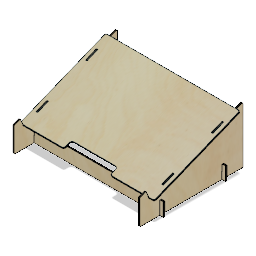
876543210 fótastandur v1 (Autodesk Fusion 360 design; units mm, degrees)
Autodesk Fusion 360 part; units mm, degrees
sketch "Sketch1" plane through (0, 0, 0) normal (1, 0, 0) x (0, 0, -1)
  line L0 (0, 0) -> (0, 55)
  line L1 (0, 55) -> (13.9078, 60.6191)
  line L2 (13.9078, 60.6191) -> (21.4942, 41.8419)
  line L3 (21.4942, 41.8419) -> (225, 124.0636)
  line L4 (225, 124.0636) -> (225, 0)
  line L5 (225, 0) -> (0, 0)
  dimension "d1" = 225
  dimension "d2" = 55
  dimension "d3" = 15
  dimension "d4" = 22
  constraint coincident L0.start L5.end
  constraint vertical L0
  constraint vertical L4
  constraint perpendicular L0 L5
  constraint parallel L1 L3
  constraint perpendicular L2 L3
  measures "d1" distance of L0.start L4.end
  measures "d2" distance of L0.start L0.end
  measures "d3" distance of L0.end L1.end
  measures "d4" angle of L3 L5
extrude "Extrude1" add sketch "Sketch1" along normal blind 2.9 makes body 1
fillet "Fillet1" radius 3 4 edges at (1.45, 55, 0) (1.45, 0, 0) (1.45, 124.0636, -225) (1.45, 0, -225) on bodies 1
fillet "Fillet2" radius 2 2 edges at (1.45, 60.6191, -13.9078) (1.45, 41.8419, -21.4942) on bodies 1
copy_body "Body->Comp2" bodies 1 removing the originals makes body 2 in component "fótur"
sketch "Sketch3" plane through (0, 28.5047, 11.5166) normal (0, 0.927184, 0.374607) x (1, 0, 0)
  line L0 (47.7026, 37.6034) -> (50.6026, 37.6034)
  line L1 (50.6026, 37.6034) -> (50.6026, 250.6437)
  line L2 (50.6026, 250.6437) -> (47.7026, 250.6437)
  line L3 (47.7026, 250.6437) -> (47.7026, 37.6034)
  line L4 (-225.1974, 37.6034) -> (-222.2974, 37.6034)
  line L5 (-222.2974, 37.6034) -> (-222.2974, 250.6437)
  line L6 (-222.2974, 250.6437) -> (-225.1974, 250.6437)
  line L7 (-225.1974, 250.6437) -> (-225.1974, 37.6034)
  line L8 (-233.1974, 238.6437) -> (58.6026, 238.6437)
  line L9 (58.6026, 238.6437) -> (58.6026, 37.6034)
  line L10 (58.6026, 37.6034) -> (-233.1974, 37.6034)
  line L11 (-233.1974, 37.6034) -> (-233.1974, 238.6437)
  line L12 (-87.2974, 238.6437) -> (-87.2974, 37.6034) construction
  line L13 (-233.1974, 138.1235) -> (58.6026, 138.1235) construction
  line L14 (-225.1974, 208.6437) -> (-222.2974, 208.6437)
  line L15 (-222.2974, 208.6437) -> (-222.2974, 183.6437)
  line L16 (-222.2974, 183.6437) -> (-225.1974, 183.6437)
  line L17 (-225.1974, 183.6437) -> (-225.1974, 208.6437)
  line L18 (-225.1974, 205.8348) -> (-225.1974, 2.7816)
  line L19 (-222.2974, 2.7816) -> (-222.2974, 205.8348)
  line L20 (50.6026, 208.6437) -> (47.7026, 208.6437)
  line L21 (47.7026, 183.6437) -> (50.6026, 183.6437)
  line L22 (50.6026, 183.6437) -> (50.6026, 208.6437)
  line L23 (47.7026, 208.6437) -> (47.7026, 183.6437)
  line L24 (-225.1974, 67.6034) -> (-222.2974, 67.6034)
  line L25 (-222.2974, 92.6034) -> (-225.1974, 92.6034)
  line L26 (-222.2974, 67.6034) -> (-222.2974, 92.6034)
  line L27 (-225.1974, 92.6034) -> (-225.1974, 67.6034)
  line L28 (50.6026, 67.6034) -> (47.7026, 67.6034)
  line L29 (47.7026, 67.6034) -> (47.7026, 92.6034)
  line L30 (50.6026, 92.6034) -> (50.6026, 67.6034)
  line L31 (47.7026, 92.6034) -> (50.6026, 92.6034)
  dimension "d42" = 8
  dimension "d43" = 8
  dimension "d44" = 12
  dimension "d45" = 25
  dimension "d46" = 30
  constraint horizontal L8
  constraint vertical L9
  constraint horizontal L10
  constraint vertical L11
  constraint collinear L0 L10
  constraint midpoint L8 L12.start
  constraint midpoint L10 L12.end
  constraint midpoint L11 L13.start
  constraint midpoint L9 L13.end
  constraint horizontal L14
  constraint vertical L15
  constraint horizontal L16
  constraint vertical L17
  constraint coincident L5 L15.end
  constraint coincident L7 L14.start
  constraint symmetric L12 L14.start L20.start
  constraint symmetric L12 L14.end L20.end
  constraint symmetric L12 L15.end L21.start
  constraint symmetric L12 L16.end L21.end
  constraint symmetric L13 L14.start L24.start
  constraint symmetric L13 L14.end L24.end
  constraint symmetric L13 L15.end L25.start
  constraint symmetric L13 L16.end L25.end
  constraint symmetric L13 L20.start L28.start
  constraint symmetric L13 L20.end L28.end
  constraint symmetric L13 L21.start L29.end
  constraint symmetric L13 L21.end L30.start
  measures "d42" distance of L7 L11
  measures "d43" distance of L1 L9
  measures "d44" distance of L1.end L8
  measures "d45" distance of L14 L16
  measures "d46" distance of L8 L14
extrude "Extrude1'" add sketch "Sketch3" against normal blind 2.9 separate body contours L0 L1 L3 L10 L28 | L3 L5 L8 L10 L15 L19 L23 L26 L29 | L1 L8 L9 L10 L22 L30 | L4 L5 L7 L10 L18 L19 L24 | L1 L3 L21 L31 | L7 L8 L10 L11 L17 L18 L27 | L5 L7 L16 L18 L19 L25 | L1 L3 L8 L20 | L5 L7 L8 L14 makes body 3 in component "Top"
combine "Combine1" operation cut target body 2 tool bodies 3 body 3 seen with x (1, 0, 0) y (0, 1, 0) z (0, 0, 1) at (-47.7026, 0, 0) keep tools in component "fótur"
combine "Combine2" operation cut target body 2 tool bodies 3 body 3 seen with x (1, 0, 0) y (0, 1, 0) z (0, 0, 1) at (225.1974, 0, 0) keep tools in component "fótur"
fillet "Fillet1'" radius 4 4 edges at (58.6026, 41.2467, -23.8918) (58.6026, 116.5577, -210.2932) (-233.1974, 116.5577, -210.2932) (-233.1974, 41.2467, -23.8918) on bodies 3 in component "Top"
fillet "Fillet1''" radius 1 5 edges at (1.45, 42.5911, -23.3486) (1.45, 53.8293, -51.1641) (1.45, 63.1945, -74.3437) (1.45, 97.2988, -158.7549) (1.45, 106.664, -181.9345) on bodies 2 in component "fótur"
ref_plane "WorkPlane1" through (49.1526, 61.3079, -180) normal (0, 0, -1) x (0, 1, 0)
sketch "Sketch5" plane through (50.8776, 60.8254, -180) normal (0, 0, -1) x (1, 0, 0)
  line L0 (-273.175, -45.057) -> (-273.175, 60.8254)
  line L1 (-273.175, 60.8254) -> (-276.075, 60.8254)
  line L2 (-276.075, 60.8254) -> (-276.075, -45.057)
  line L3 (-0.275, -45.057) -> (-0.275, 60.8254)
  line L4 (-0.275, 60.8254) -> (-3.175, 60.8254)
  line L5 (-3.175, 60.8254) -> (-3.175, -45.057)
  line L6 (7.725, 30.8254) -> (-284.075, 30.8254)
  line L7 (-284.075, 30.8254) -> (-284.075, 60.8254)
  line L8 (-284.075, 60.8254) -> (7.725, 60.8254)
  line L9 (7.725, 60.8254) -> (7.725, 30.8254)
  line L10 (7.725, -52.8895) -> (7.725, 19.4247)
  line L11 (-284.075, 19.4247) -> (-284.075, -52.8895)
  line L12 (-0.275, 30.8254) -> (-3.175, 30.8254)
  line L13 (-3.175, 30.8254) -> (-3.175, 45.8254)
  line L14 (-3.175, 45.8254) -> (-0.275, 45.8254)
  line L15 (-0.275, 45.8254) -> (-0.275, 30.8254)
  line L16 (-276.075, 30.8254) -> (-273.175, 30.8254)
  line L17 (-273.175, 30.8254) -> (-273.175, 45.8254)
  line L18 (-273.175, 45.8254) -> (-276.075, 45.8254)
  line L19 (-276.075, 45.8254) -> (-276.075, 30.8254)
  line L20 (-276.075, -45.057) -> (-273.175, -45.057)
  line L21 (-3.175, -45.057) -> (-0.275, -45.057)
  dimension "d55" = 30
  dimension "d56" = 15
  dimension "d57" = 15
  constraint horizontal L6
  constraint vertical L7
  constraint horizontal L8
  constraint vertical L9
  constraint collinear L1 L8
  constraint collinear L9 L10
  constraint collinear L7 L11
  constraint horizontal L12
  constraint vertical L13
  constraint horizontal L14
  constraint vertical L15
  constraint coincident L5 L13.end
  constraint coincident L6 L12.start
  constraint coincident L3 L12.start
  constraint horizontal L16
  constraint vertical L17
  constraint horizontal L18
  constraint vertical L19
  constraint coincident L0 L17.end
  constraint coincident L2 L16.start
  constraint coincident L6 L16.start
  measures "d55" distance of L6 L8
  measures "d56" distance of L6 L14
  measures "d57" distance of L6 L18
extrude "Extrude2" add sketch "Sketch5" along normal mid plane 2.9 separate body contours L0 L5 L6 L8 L13 L17 | L0 L1 L2 L8 L18 | L2 L6 L7 L8 L19 | L3 L4 L5 L8 L14 | L3 L6 L8 L9 L15 makes body 4
ref_plane "WorkPlane2" through (49.1526, 27.9882, -112.5) normal (0, 0, 1) x (0, -1, 0)
mirror "Mirror1" about plane through (49.1526, 27.9882, -112.5) normal (0, 0, 1) of bodies 4 makes body 5
combine "Combine3" operation cut target body 2 tool bodies 4 5 body 4 seen with x (1, 0, 0) y (0, 1, 0) z (0, 0, 1) at (-47.7026, 0, 0) body 5 seen with x (1, 0, 0) y (0, 1, 0) z (0, 0, 1) at (-47.7026, 0, 0) keep tools in component "fótur"
combine "Combine4" operation cut target body 2 tool bodies 4 5 body 4 seen with x (1, 0, 0) y (0, 1, 0) z (0, 0, 1) at (225.1974, 0, 0) body 5 seen with x (1, 0, 0) y (0, 1, 0) z (0, 0, 1) at (225.1974, 0, 0) keep tools in component "fótur"
fillet "Fillet3" radius 1 12 edges at (50.6026, 30, -180) (47.7026, 30, -180) (58.6026, 30, -180) (-222.2974, 30, -180) (-225.1974, 30, -180) (-233.1974, 30, -180) (50.6026, 30, -45) (47.7026, 30, -45) (-222.2974, 30, -45) (-225.1974, 30, -45) (-233.1974, 30, -45) (58.6026, 30, -45) on bodies 4 5
fillet "Fillet2'" radius 1 4 edges at (1.45, 0, -43.55) (1.45, 0, -46.45) (1.45, 0, -178.55) (1.45, 0, -181.45) on bodies 2 in component "fótur"
sketch "Sketch6" plane through (0, 28.5047, 11.5166) normal (0, 0.927184, 0.374607) x (1, 0, 0)
  arc A0 (-233.1974, 41.6034) -> (-229.1974, 37.6034) centre (-229.1974, 41.6034) ccw
  line L0 (-229.1974, 37.6034) -> (54.6026, 37.6034)
  arc A1 (54.6026, 37.6034) -> (58.6026, 41.6034) centre (54.6026, 41.6034) ccw
  line L1 (58.6026, 41.6034) -> (58.6026, 234.6437)
  arc A2 (58.6026, 234.6437) -> (54.6026, 238.6437) centre (54.6026, 234.6437) ccw
  line L2 (54.6026, 238.6437) -> (-229.1974, 238.6437)
  arc A3 (-229.1974, 238.6437) -> (-233.1974, 234.6437) centre (-229.1974, 234.6437) ccw
  line L3 (-233.1974, 234.6437) -> (-233.1974, 41.6034)
  line L4 (47.7026, 67.6034) -> (47.7026, 92.6034)
  line L5 (47.7026, 92.6034) -> (50.6026, 92.6034)
  line L6 (50.6026, 92.6034) -> (50.6026, 67.6034)
  line L7 (50.6026, 67.6034) -> (47.7026, 67.6034)
  line L8 (-225.1974, 183.6437) -> (-225.1974, 208.6437)
  line L9 (-225.1974, 208.6437) -> (-222.2974, 208.6437)
  line L10 (-222.2974, 208.6437) -> (-222.2974, 183.6437)
  line L11 (-222.2974, 183.6437) -> (-225.1974, 183.6437)
  line L12 (-225.1974, 67.6034) -> (-225.1974, 92.6034)
  line L13 (-225.1974, 92.6034) -> (-222.2974, 92.6034)
  line L14 (-222.2974, 92.6034) -> (-222.2974, 67.6034)
  line L15 (-222.2974, 67.6034) -> (-225.1974, 67.6034)
  line L16 (47.7026, 183.6437) -> (47.7026, 208.6437)
  line L17 (47.7026, 208.6437) -> (50.6026, 208.6437)
  line L18 (50.6026, 208.6437) -> (50.6026, 183.6437)
  line L19 (50.6026, 183.6437) -> (47.7026, 183.6437)
  line L20 (-229.1974, 238.6437) -> (54.6026, 238.6437)
  line L21 (54.6026, 37.6034) -> (-229.1974, 37.6034)
  line L22 (-137.2974, 55.1034) -> (-37.2974, 55.1034)
  line L23 (-37.2974, 55.1034) -> (-37.2974, 20.1034)
  line L24 (-37.2974, 20.1034) -> (-137.2974, 20.1034)
  line L25 (-137.2974, 20.1034) -> (-137.2974, 55.1034)
  line L26 (-137.2974, 55.1034) -> (-37.2974, 20.1034) construction
  line L27 (-37.2974, 55.1034) -> (-137.2974, 20.1034) construction
  point P0 (-87.2974, 37.6034)
  dimension "d64" = 100
  dimension "d65" = 35
  constraint perpendicular L22 L23
  constraint parallel L22 L24
  constraint parallel L23 L25
  constraint horizontal L22
  constraint coincident L26 P0
  constraint coincident L27 P0
  constraint midpoint L21 P0
  measures "d64" distance of L23.end L24.end
  measures "d65" distance of L22.end L23.end
extrude "Extrude2'" cut sketch "Sketch6" against normal up to surface (2.9 mm away) contours L0 L21 L22 L23 L25 bodies 3 in component "Top"
fillet "Fillet2''" radius 5 4 edges at (-37.2974, 47.8023, -40.1175) (-37.2974, 41.2467, -23.8918) (-137.2974, 47.8023, -40.1175) (-137.2974, 41.2467, -23.8918) on bodies 3 in component "Top"
sketch "Sketch10" plane through (50.6026, 0, 0) normal (1, 0, 0) x (0, 0, -1)
  arc A0 (181.45, 1) -> (182.45, 0) centre (182.45, 1) ccw
  line L0 (182.45, 0) -> (222, 0)
  arc A1 (222, 0) -> (225, 3) centre (222, 3) ccw
  line L1 (225, 3) -> (225, 119.6159)
  arc A2 (225, 119.6159) -> (220.8762, 122.3974) centre (222, 119.6159) ccw
  line L2 (220.8762, 122.3974) -> (209.75, 117.9022)
  line L3 (209.75, 117.9022) -> (210.8363, 115.2133)
  line L4 (210.8363, 115.2133) -> (183.0208, 103.9751)
  line L5 (183.0208, 103.9751) -> (182.3091, 105.7368)
  arc A3 (182.3091, 105.7368) -> (181.0073, 106.2894) centre (181.3819, 105.3622) ccw
  line L6 (181.0073, 106.2894) -> (159.682, 97.6734)
  arc A4 (159.682, 97.6734) -> (159.1295, 96.3716) centre (160.0567, 96.7462) ccw
  line L7 (159.1295, 96.3716) -> (159.8412, 94.61)
  line L8 (159.8412, 94.61) -> (75.4301, 60.5056)
  line L9 (75.4301, 60.5056) -> (74.7183, 62.2673)
  arc A5 (74.7183, 62.2673) -> (73.4165, 62.8199) centre (73.7911, 61.8927) ccw
  line L10 (73.4165, 62.8199) -> (52.0913, 54.2039)
  arc A6 (52.0913, 54.2039) -> (51.5387, 52.9021) centre (52.4659, 53.2767) ccw
  line L11 (51.5387, 52.9021) -> (52.2505, 51.1405)
  line L12 (52.2505, 51.1405) -> (24.435, 39.9023)
  line L13 (24.435, 39.9023) -> (23.6589, 41.823)
  arc A7 (23.6589, 41.823) -> (22.6876, 42.4474) centre (22.7318, 41.4484) ccw
  arc A8 (20.745, 43.6963) -> (22.6876, 42.4474) centre (22.5994, 44.4455) ccw
  line L14 (20.745, 43.6963) -> (14.657, 58.7647)
  arc A9 (14.657, 58.7647) -> (12.0534, 59.8699) centre (12.8026, 58.0155) ccw
  line L15 (12.0534, 59.8699) -> (1.8762, 55.758)
  arc A10 (1.8762, 55.758) -> (0, 52.9765) centre (3, 52.9765) ccw
  line L16 (0, 52.9765) -> (0, 3)
  arc A11 (0, 3) -> (3, 0) centre (3, 3) ccw
  line L17 (3, 0) -> (42.55, 0)
  arc A12 (42.55, 0) -> (43.55, 1) centre (42.55, 1) ccw
  line L18 (43.55, 1) -> (43.55, 15)
  line L19 (43.55, 15) -> (46.45, 15)
  line L20 (46.45, 15) -> (46.45, 1)
  arc A13 (46.45, 1) -> (47.45, 0) centre (47.45, 1) ccw
  line L21 (47.45, 0) -> (177.55, 0)
  arc A14 (177.55, 0) -> (178.55, 1) centre (177.55, 1) ccw
  line L22 (178.55, 1) -> (178.55, 15)
  line L23 (178.55, 15) -> (181.45, 15)
  line L24 (181.45, 15) -> (181.45, 1)
sketch "Top_DXF" plane through (0, 28.5047, 11.5166) normal (0, 0.927184, 0.374607) x (1, 0, 0)
  line L0 (47.7026, 67.6034) -> (47.7026, 92.6034)
  line L1 (47.7026, 92.6034) -> (50.6026, 92.6034)
  line L2 (50.6026, 92.6034) -> (50.6026, 67.6034)
  line L3 (50.6026, 67.6034) -> (47.7026, 67.6034)
  line L4 (-225.1974, 183.6437) -> (-225.1974, 208.6437)
  line L5 (-225.1974, 208.6437) -> (-222.2974, 208.6437)
  line L6 (-222.2974, 208.6437) -> (-222.2974, 183.6437)
  line L7 (-222.2974, 183.6437) -> (-225.1974, 183.6437)
  line L8 (-225.1974, 67.6034) -> (-225.1974, 92.6034)
  line L9 (-225.1974, 92.6034) -> (-222.2974, 92.6034)
  line L10 (-222.2974, 92.6034) -> (-222.2974, 67.6034)
  line L11 (-222.2974, 67.6034) -> (-225.1974, 67.6034)
  line L12 (47.7026, 183.6437) -> (47.7026, 208.6437)
  line L13 (47.7026, 208.6437) -> (50.6026, 208.6437)
  line L14 (50.6026, 208.6437) -> (50.6026, 183.6437)
  line L15 (50.6026, 183.6437) -> (47.7026, 183.6437)
  arc A0 (-142.2974, 37.6034) -> (-137.2974, 42.6034) centre (-142.2974, 42.6034) ccw
  line L16 (-137.2974, 42.6034) -> (-137.2974, 50.1034)
  arc A1 (-132.2974, 55.1034) -> (-137.2974, 50.1034) centre (-132.2974, 50.1034) ccw
  line L17 (-132.2974, 55.1034) -> (-42.2974, 55.1034)
  arc A2 (-37.2974, 50.1034) -> (-42.2974, 55.1034) centre (-42.2974, 50.1034) ccw
  line L18 (-37.2974, 50.1034) -> (-37.2974, 42.6034)
  arc A3 (-37.2974, 42.6034) -> (-32.2974, 37.6034) centre (-32.2974, 42.6034) ccw
  line L19 (-32.2974, 37.6034) -> (54.6026, 37.6034)
  arc A4 (54.6026, 37.6034) -> (58.6026, 41.6034) centre (54.6026, 41.6034) ccw
  line L20 (58.6026, 41.6034) -> (58.6026, 234.6437)
  arc A5 (58.6026, 234.6437) -> (54.6026, 238.6437) centre (54.6026, 234.6437) ccw
  line L21 (54.6026, 238.6437) -> (-229.1974, 238.6437)
  arc A6 (-229.1974, 238.6437) -> (-233.1974, 234.6437) centre (-229.1974, 234.6437) ccw
  line L22 (-233.1974, 234.6437) -> (-233.1974, 41.6034)
  arc A7 (-233.1974, 41.6034) -> (-229.1974, 37.6034) centre (-229.1974, 41.6034) ccw
  line L23 (-229.1974, 37.6034) -> (-142.2974, 37.6034)
sketch "Support_DXF" plane through (0, 0, -43.55) normal (0, 0, 1) x (1, 0, 0)
  arc A0 (58.6026, 29) -> (57.6026, 30) centre (57.6026, 29) ccw
  line L0 (57.6026, 30) -> (51.6026, 30)
  arc A1 (51.6026, 30) -> (50.6026, 29) centre (51.6026, 29) ccw
  line L1 (50.6026, 29) -> (50.6026, 15)
  line L2 (50.6026, 15) -> (47.7026, 15)
  line L3 (47.7026, 15) -> (47.7026, 29)
  arc A2 (47.7026, 29) -> (46.7026, 30) centre (46.7026, 29) ccw
  line L4 (46.7026, 30) -> (-221.2974, 30)
  arc A3 (-221.2974, 30) -> (-222.2974, 29) centre (-221.2974, 29) ccw
  line L5 (-222.2974, 29) -> (-222.2974, 15)
  line L6 (-222.2974, 15) -> (-225.1974, 15)
  line L7 (-225.1974, 15) -> (-225.1974, 29)
  arc A4 (-225.1974, 29) -> (-226.1974, 30) centre (-226.1974, 29) ccw
  line L8 (-226.1974, 30) -> (-232.1974, 30)
  arc A5 (-232.1974, 30) -> (-233.1974, 29) centre (-232.1974, 29) ccw
  line L9 (-233.1974, 29) -> (-233.1974, 0)
  line L10 (-233.1974, 0) -> (58.6026, 0)
  line L11 (58.6026, 0) -> (58.6026, 29)
sketch "Leg_DXF" plane through (50.6026, 0, 0) normal (1, 0, 0) x (0, 0, -1)
  arc A0 (181.45, 1) -> (182.45, 0) centre (182.45, 1) ccw
  line L0 (182.45, 0) -> (222, 0)
  arc A1 (222, 0) -> (225, 3) centre (222, 3) ccw
  line L1 (225, 3) -> (225, 119.6159)
  arc A2 (225, 119.6159) -> (220.8762, 122.3974) centre (222, 119.6159) ccw
  line L2 (220.8762, 122.3974) -> (209.75, 117.9022)
  line L3 (209.75, 117.9022) -> (210.8363, 115.2133)
  line L4 (210.8363, 115.2133) -> (183.0208, 103.9751)
  line L5 (183.0208, 103.9751) -> (182.3091, 105.7368)
  arc A3 (182.3091, 105.7368) -> (181.0073, 106.2894) centre (181.3819, 105.3622) ccw
  line L6 (181.0073, 106.2894) -> (159.682, 97.6734)
  arc A4 (159.682, 97.6734) -> (159.1295, 96.3716) centre (160.0567, 96.7462) ccw
  line L7 (159.1295, 96.3716) -> (159.8412, 94.61)
  line L8 (159.8412, 94.61) -> (75.4301, 60.5056)
  line L9 (75.4301, 60.5056) -> (74.7183, 62.2673)
  arc A5 (74.7183, 62.2673) -> (73.4165, 62.8199) centre (73.7911, 61.8927) ccw
  line L10 (73.4165, 62.8199) -> (52.0913, 54.2039)
  arc A6 (52.0913, 54.2039) -> (51.5387, 52.9021) centre (52.4659, 53.2767) ccw
  line L11 (51.5387, 52.9021) -> (52.2505, 51.1405)
  line L12 (52.2505, 51.1405) -> (24.435, 39.9023)
  line L13 (24.435, 39.9023) -> (23.6589, 41.823)
  arc A7 (23.6589, 41.823) -> (22.6876, 42.4474) centre (22.7318, 41.4484) ccw
  arc A8 (20.745, 43.6963) -> (22.6876, 42.4474) centre (22.5994, 44.4455) ccw
  line L14 (20.745, 43.6963) -> (14.657, 58.7647)
  arc A9 (14.657, 58.7647) -> (12.0534, 59.8699) centre (12.8026, 58.0155) ccw
  line L15 (12.0534, 59.8699) -> (1.8762, 55.758)
  arc A10 (1.8762, 55.758) -> (0, 52.9765) centre (3, 52.9765) ccw
  line L16 (0, 52.9765) -> (0, 3)
  arc A11 (0, 3) -> (3, 0) centre (3, 3) ccw
  line L17 (3, 0) -> (42.55, 0)
  arc A12 (42.55, 0) -> (43.55, 1) centre (42.55, 1) ccw
  line L18 (43.55, 1) -> (43.55, 15)
  line L19 (43.55, 15) -> (46.45, 15)
  line L20 (46.45, 15) -> (46.45, 1)
  arc A13 (46.45, 1) -> (47.45, 0) centre (47.45, 1) ccw
  line L21 (47.45, 0) -> (177.55, 0)
  arc A14 (177.55, 0) -> (178.55, 1) centre (177.55, 1) ccw
  line L22 (178.55, 1) -> (178.55, 15)
  line L23 (178.55, 15) -> (181.45, 15)
  line L24 (181.45, 15) -> (181.45, 1)
fillet "Fillet4" radius 0.2 84 edges at (49.1526, 15, -181.45) (49.1526, 15, -178.55) (-222.2974, 15, -180) (50.6026, 15, -180) (47.7026, 15, -180) (-223.7474, 15, -178.55) (-225.1974, 15, -180) (-87.2974, 0, -178.55) (-87.2974, 0, -181.45) (47.7026, 22, -178.55) (47.4097, 29.7071, -178.55) (-87.2974, 30, -178.55) (-222.0045, 29.7071, -178.55) (-222.2974, 22, -178.55) (-222.2974, 22, -181.45) (-222.0045, 29.7071, -181.45) (-87.2974, 30, -181.45) (47.4097, 29.7071, -181.45) (47.7026, 22, -181.45) (50.6026, 22, -181.45) (50.8955, 29.7071, -181.45) (54.6026, 30, -181.45) (58.3097, 29.7071, -181.45) (58.6026, 14.5, -181.45) (-223.7474, 15, -181.45) (58.6026, 0, -180) (58.6026, 14.5, -178.55) (58.3097, 29.7071, -178.55) (54.6026, 30, -178.55) (50.8955, 29.7071, -178.55) (50.6026, 22, -178.55) (-233.1974, 0, -180) (-233.1974, 14.5, -181.45) (-232.9045, 29.7071, -181.45) (-229.1974, 30, -181.45) (-225.4903, 29.7071, -181.45) (-225.1974, 22, -181.45) (-225.1974, 22, -178.55) (-225.4903, 29.7071, -178.55) (-229.1974, 30, -178.55) (-232.9045, 29.7071, -178.55) (-233.1974, 14.5, -178.55) (58.6026, 0, -45) (49.1526, 15, -43.55) (-233.1974, 14.5, -43.55) (-232.9045, 29.7071, -43.55) (-229.1974, 30, -43.55) (-225.4903, 29.7071, -43.55) (-225.1974, 22, -43.55) (-87.2974, 0, -46.45) (-87.2974, 0, -43.55) (47.7026, 22, -46.45) (47.4097, 29.7071, -46.45) (-87.2974, 30, -46.45) (-222.0045, 29.7071, -46.45) (-222.2974, 22, -46.45) (-222.2974, 22, -43.55) (-222.0045, 29.7071, -43.55) (-87.2974, 30, -43.55) (47.4097, 29.7071, -43.55) (47.7026, 22, -43.55) (50.6026, 22, -43.55) (50.8955, 29.7071, -43.55) (54.6026, 30, -43.55) (58.3097, 29.7071, -43.55) (58.6026, 14.5, -43.55) (58.6026, 14.5, -46.45) (58.3097, 29.7071, -46.45) (54.6026, 30, -46.45) (50.8955, 29.7071, -46.45) (50.6026, 22, -46.45) (-222.2974, 15, -45) (-223.7474, 15, -46.45) (-225.1974, 15, -45) (-223.7474, 15, -43.55) (-225.1974, 22, -46.45) (-225.4903, 29.7071, -46.45) (-229.1974, 30, -46.45) (-232.9045, 29.7071, -46.45) (-233.1974, 14.5, -46.45) (-233.1974, 0, -45) (50.6026, 15, -45) (47.7026, 15, -45) (49.1526, 15, -46.45) on bodies 4 5
fillet "Fillet3'" radius 0.2 182 edges at (0, 116.5577, -210.2932) (1.45, 117.9022, -209.75) (2.9, 116.5577, -210.2932) (2.9, 8, -46.45) (2.9, 0.2929, -46.7429) (2.9, 0, -112.5) (2.9, 0.2929, -178.2571) (2.9, 8, -178.55) (2.9, 8, -181.45) (2.9, 0.2929, -181.7429) (2.9, 0, -202.225) (2.9, 0.8787, -224.1213) (2.9, 61.3079, -225) (2.9, 122.103, -223.6776) (2.9, 120.1498, -215.3131) (1.45, 39.9023, -24.435) (1.45, 60.5056, -75.4301) (1.45, 51.1405, -52.2505) (0, 120.1498, -215.3131) (0, 122.103, -223.6776) (0, 61.3079, -225) (0, 0.8787, -224.1213) (0, 0, -202.225) (0, 0.2929, -181.7429) (0, 8, -181.45) (2.9, 40.8626, -24.047) (2.9, 42.2896, -23.2725) (2.9, 42.7631, -21.5179) (2.9, 51.2305, -17.701) (2.9, 59.8565, -13.5841) (2.9, 57.814, -6.9648) (2.9, 54.6541, -0.5129) (2.9, 27.9882, 0) (2.9, 0.8787, -0.8787) (2.9, 0, -22.775) (2.9, 0.2929, -43.2571) (2.9, 8, -43.55) (1.45, 103.9751, -183.0208) (0, 8, -178.55) (0, 0.2929, -178.2571) (0, 0, -112.5) (0, 0.2929, -46.7429) (0, 8, -46.45) (0, 45.5214, -38.3427) (2.9, 77.5578, -117.6356) (0, 120.1498, -215.3131) (0, 122.103, -223.6776) (0, 61.3079, -225) (0, 0.8787, -224.1213) (0, 0, -202.225) (0, 0.2929, -181.7429) (0, 8, -181.45) (2.9, 15, -45) (0, 15, -45) (0, 95.4908, -159.4853) (0, 97.137, -159.1361) (0, 101.9814, -170.3447) (0, 106.2827, -181.7726) (0, 104.856, -182.6649) (2.9, 104.856, -182.6649) (2.9, 106.2827, -181.7726) (2.9, 101.9814, -170.3447) (2.9, 97.137, -159.1361) (2.9, 95.4908, -159.4853) (1.45, 94.61, -159.8412) (0, 52.0213, -51.8946) (0, 53.6675, -51.5454) (0, 58.5119, -62.7539) (0, 62.8132, -74.1819) (0, 61.3865, -75.0742) (2.9, 61.3865, -75.0742) (2.9, 62.8132, -74.1819) (2.9, 58.5119, -62.7539) (2.9, 53.6675, -51.5454) (2.9, 52.0213, -51.8946) (2.9, 8, -46.45) (2.9, 0.2929, -46.7429) (2.9, 0, -112.5) (2.9, 0.2929, -178.2571) (2.9, 8, -178.55) (1.45, 15, -46.45) (1.45, 15, -43.55) (2.9, 15, -45) (0, 15, -45) (0, 95.4908, -159.4853) (0, 97.137, -159.1361) (0, 101.9814, -170.3447) (0, 106.2827, -181.7726) (0, 104.856, -182.6649) (2.9, 104.856, -182.6649) (2.9, 106.2827, -181.7726) (2.9, 101.9814, -170.3447) (2.9, 97.137, -159.1361) (2.9, 95.4908, -159.4853) (1.45, 94.61, -159.8412) (1.45, 60.5056, -75.4301) (2.9, 61.3865, -75.0742) (2.9, 62.8132, -74.1819) (2.9, 58.5119, -62.7539) (2.9, 53.6675, -51.5454) (2.9, 52.0213, -51.8946) (0, 8, -43.55) (0, 0.2929, -43.2571) (0, 0, -22.775) (0, 0.8787, -0.8787) (0, 27.9882, 0) (0, 54.6541, -0.5129) (0, 57.814, -6.9648) (0, 59.8565, -13.5841) (0, 51.2305, -17.701) (0, 42.7631, -21.5179) (0, 42.2896, -23.2725) (0, 40.8626, -24.047) (1.45, 15, -46.45) (1.45, 15, -43.55) (0, 109.5942, -196.9286) (2.9, 109.5942, -196.9286) (1.45, 115.2133, -210.8363) (1.45, 15, -178.55) (1.45, 15, -181.45) (2.9, 15, -180) (0, 15, -180) (2.9, 77.5578, -117.6356) (0, 77.5578, -117.6356) (2.9, 8, -181.45) (2.9, 0.2929, -181.7429) (2.9, 0, -202.225) (2.9, 0.8787, -224.1213) (2.9, 61.3079, -225) (2.9, 122.103, -223.6776) (2.9, 120.1498, -215.3131) (1.45, 103.9751, -183.0208) (0, 116.5577, -210.2932) (1.45, 117.9022, -209.75) (2.9, 116.5577, -210.2932) (0, 109.5942, -196.9286) (2.9, 109.5942, -196.9286) (1.45, 115.2133, -210.8363) (1.45, 15, -178.55) (1.45, 15, -181.45) (2.9, 15, -180) (0, 45.5214, -38.3427) (2.9, 45.5214, -38.3427) (0, 77.5578, -117.6356) (0, 15, -180) (0, 52.0213, -51.8946) (0, 53.6675, -51.5454) (0, 58.5119, -62.7539) (0, 62.8132, -74.1819) (0, 61.3865, -75.0742) (1.45, 39.9023, -24.435) (1.45, 51.1405, -52.2505) (2.9, 40.8626, -24.047) (2.9, 42.2896, -23.2725) (2.9, 42.7631, -21.5179) (2.9, 51.2305, -17.701) (2.9, 59.8565, -13.5841) (2.9, 57.814, -6.9648) (2.9, 54.6541, -0.5129) (2.9, 27.9882, 0) (2.9, 0.8787, -0.8787) (2.9, 0, -22.775) (2.9, 0.2929, -43.2571) (2.9, 8, -43.55) (0, 8, -43.55) (0, 0.2929, -43.2571) (0, 0, -22.775) (0, 0.8787, -0.8787) (0, 27.9882, 0) (0, 54.6541, -0.5129) (0, 57.814, -6.9648) (0, 59.8565, -13.5841) (0, 51.2305, -17.701) (0, 42.7631, -21.5179) (0, 42.2896, -23.2725) (0, 40.8626, -24.047) (2.9, 45.5214, -38.3427) (0, 8, -178.55) (0, 0.2929, -178.2571) (0, 0, -112.5) (0, 0.2929, -46.7429) (0, 8, -46.45) on bodies 2 in component "fótur"
fillet "Fillet3''" radius 0.2 80 edges at (50.6026, 58.5119, -62.7539) (-37.2974, 45.8689, -31.4615) (-38.7619, 48.5981, -38.2165) (-87.2974, 49.1467, -39.5743) (-135.8329, 48.5981, -38.2165) (-137.2974, 45.8689, -31.4615) (-138.7619, 43.1397, -24.7064) (-185.7474, 42.5911, -23.3486) (-232.0258, 43.03, -24.4349) (-233.1974, 80.2466, -116.5493) (-232.0258, 117.4633, -208.6637) (-87.2974, 117.9022, -209.75) (57.431, 117.4633, -208.6637) (58.6026, 80.2466, -116.5493) (57.431, 43.03, -24.4349) (11.1526, 42.5911, -23.3486) (-35.8329, 43.1397, -24.7064) (49.1526, 63.1945, -74.3437) (-35.8329, 40.4509, -25.7928) (-37.2974, 43.1801, -32.5478) (-38.7619, 45.9093, -39.3029) (-87.2974, 46.4579, -40.6607) (-135.8329, 45.9093, -39.3029) (-137.2974, 43.1801, -32.5478) (-138.7619, 40.4509, -25.7928) (-185.7474, 39.9023, -24.435) (-232.0258, 40.3412, -25.5212) (-233.1974, 77.5578, -117.6356) (-232.0258, 114.7744, -209.7501) (-87.2974, 115.2133, -210.8363) (57.431, 114.7744, -209.7501) (58.6026, 77.5578, -117.6356) (57.431, 40.3412, -25.5212) (11.1526, 39.9023, -24.435) (49.1526, 106.664, -181.9345) (50.6026, 101.9814, -170.3447) (47.7026, 105.3195, -182.4776) (50.6026, 105.3195, -182.4776) (49.1526, 97.2988, -158.7549) (50.6026, 95.9544, -159.298) (49.1526, 103.9751, -183.0208) (47.7026, 101.9814, -170.3447) (49.1526, 60.5056, -75.4301) (47.7026, 58.5119, -62.7539) (47.7026, 95.9544, -159.298) (50.6026, 99.2925, -171.431) (47.7026, 99.2925, -171.431) (50.6026, 55.8231, -63.8403) (50.6026, 52.4849, -51.7073) (-223.7474, 53.8293, -51.1641) (-223.7474, 51.1405, -52.2505) (-223.7474, 60.5056, -75.4301) (-222.2974, 58.5119, -62.7539) (-225.1974, 52.4849, -51.7073) (-225.1974, 61.8501, -74.8869) (-222.2974, 61.8501, -74.8869) (-222.2974, 55.8231, -63.8403) (-222.2974, 52.4849, -51.7073) (-225.1974, 58.5119, -62.7539) (-225.1974, 55.8231, -63.8403) (-223.7474, 63.1945, -74.3437) (-223.7474, 106.664, -181.9345) (-222.2974, 101.9814, -170.3447) (-225.1974, 105.3195, -182.4776) (-222.2974, 105.3195, -182.4776) (-223.7474, 97.2988, -158.7549) (-222.2974, 95.9544, -159.298) (-223.7474, 103.9751, -183.0208) (-225.1974, 101.9814, -170.3447) (-225.1974, 95.9544, -159.298) (-222.2974, 99.2925, -171.431) (-225.1974, 99.2925, -171.431) (-223.7474, 94.61, -159.8412) (49.1526, 94.61, -159.8412) (49.1526, 53.8293, -51.1641) (49.1526, 51.1405, -52.2505) (47.7026, 52.4849, -51.7073) (47.7026, 61.8501, -74.8869) (50.6026, 61.8501, -74.8869) (47.7026, 55.8231, -63.8403) on bodies 3 in component "Top"
sketch "Sketch11" plane through (0, 28.5047, 11.5166) normal (0, 0.927184, 0.374607) x (1, 0, 0)
  arc A0 (-222.4974, 67.4034) -> (-222.0974, 67.8034) centre (-222.4974, 67.8034) ccw
  line L0 (-222.4974, 67.4034) -> (-224.9974, 67.4034)
  arc A1 (-225.3974, 67.8034) -> (-224.9974, 67.4034) centre (-224.9974, 67.8034) ccw
  line L1 (-225.3974, 67.8034) -> (-225.3974, 92.4034)
  arc A2 (-224.9974, 92.8034) -> (-225.3974, 92.4034) centre (-224.9974, 92.4034) ccw
  line L2 (-224.9974, 92.8034) -> (-222.4974, 92.8034)
  arc A3 (-222.0974, 92.4034) -> (-222.4974, 92.8034) centre (-222.4974, 92.4034) ccw
  line L3 (-222.0974, 92.4034) -> (-222.0974, 67.8034)
  line L4 (-37.0974, 50.1034) -> (-37.0974, 42.6034)
  arc A4 (-37.0974, 42.6034) -> (-32.2974, 37.8034) centre (-32.2974, 42.6034) ccw
  line L5 (-32.2974, 37.8034) -> (54.6026, 37.8034)
  arc A5 (54.6026, 37.8034) -> (58.4026, 41.6034) centre (54.6026, 41.6034) ccw
  line L6 (58.4026, 41.6034) -> (58.4026, 234.6437)
  arc A6 (58.4026, 234.6437) -> (54.6026, 238.4437) centre (54.6026, 234.6437) ccw
  line L7 (54.6026, 238.4437) -> (-229.1974, 238.4437)
  arc A7 (-229.1974, 238.4437) -> (-232.9974, 234.6437) centre (-229.1974, 234.6437) ccw
  line L8 (-232.9974, 234.6437) -> (-232.9974, 41.6034)
  arc A8 (-232.9974, 41.6034) -> (-229.1974, 37.8034) centre (-229.1974, 41.6034) ccw
  line L9 (-229.1974, 37.8034) -> (-142.2974, 37.8034)
  arc A9 (-142.2974, 37.8034) -> (-137.4974, 42.6034) centre (-142.2974, 42.6034) ccw
  line L10 (-137.4974, 42.6034) -> (-137.4974, 50.1034)
  arc A10 (-132.2974, 55.3034) -> (-137.4974, 50.1034) centre (-132.2974, 50.1034) ccw
  line L11 (-132.2974, 55.3034) -> (-42.2974, 55.3034)
  arc A11 (-37.0974, 50.1034) -> (-42.2974, 55.3034) centre (-42.2974, 50.1034) ccw
  arc A12 (50.8026, 92.4034) -> (50.4026, 92.8034) centre (50.4026, 92.4034) ccw
  line L12 (50.8026, 92.4034) -> (50.8026, 67.8034)
  arc A13 (50.4026, 67.4034) -> (50.8026, 67.8034) centre (50.4026, 67.8034) ccw
  line L13 (50.4026, 67.4034) -> (47.9026, 67.4034)
  arc A14 (47.5026, 67.8034) -> (47.9026, 67.4034) centre (47.9026, 67.8034) ccw
  line L14 (47.5026, 67.8034) -> (47.5026, 92.4034)
  arc A15 (47.9026, 92.8034) -> (47.5026, 92.4034) centre (47.9026, 92.4034) ccw
  line L15 (47.9026, 92.8034) -> (50.4026, 92.8034)
  arc A16 (47.9026, 208.8437) -> (47.5026, 208.4437) centre (47.9026, 208.4437) ccw
  line L16 (47.9026, 208.8437) -> (50.4026, 208.8437)
  arc A17 (50.8026, 208.4437) -> (50.4026, 208.8437) centre (50.4026, 208.4437) ccw
  line L17 (50.8026, 208.4437) -> (50.8026, 183.8437)
  arc A18 (50.4026, 183.4437) -> (50.8026, 183.8437) centre (50.4026, 183.8437) ccw
  line L18 (50.4026, 183.4437) -> (47.9026, 183.4437)
  arc A19 (47.5026, 183.8437) -> (47.9026, 183.4437) centre (47.9026, 183.8437) ccw
  line L19 (47.5026, 183.8437) -> (47.5026, 208.4437)
  arc A20 (-224.9974, 208.8437) -> (-225.3974, 208.4437) centre (-224.9974, 208.4437) ccw
  line L20 (-224.9974, 208.8437) -> (-222.4974, 208.8437)
  arc A21 (-222.0974, 208.4437) -> (-222.4974, 208.8437) centre (-222.4974, 208.4437) ccw
  line L21 (-222.0974, 208.4437) -> (-222.0974, 183.8437)
  arc A22 (-222.4974, 183.4437) -> (-222.0974, 183.8437) centre (-222.4974, 183.8437) ccw
  line L22 (-222.4974, 183.4437) -> (-224.9974, 183.4437)
  arc A23 (-225.3974, 183.8437) -> (-224.9974, 183.4437) centre (-224.9974, 183.8437) ccw
  line L23 (-225.3974, 183.8437) -> (-225.3974, 208.4437)
component "fótur" placed x (1, 0, 0) y (0, 1, 0) z (0, 0, 1) at (-225.1974, 0, 0)
component "fótur" placed x (1, 0, 0) y (0, 1, 0) z (0, 0, 1) at (47.7026, 0, 0)
component "Top" placed x (1, 0, 0) y (0, 1, 0) z (0, 0, 1) at (0, 0, 0)
equation "efnisþykkt = 2.9 mm"
equation "fótaþykkt = 270 mm"
equation "d7 = efnisþykkt"
equation "d30 = fótaþykkt"
equation "d47 = -efnisþykkt"
equation "d58 = efnisþykkt / 2"
equation "toppslengd = 291.40 mm"
named bodies: "Support", "Support (1)"
